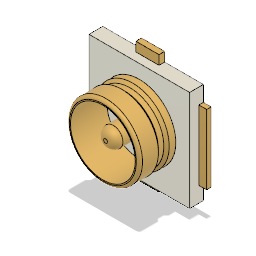
U.FL_Molex_MCRF_73412-0110_Vertical (Autodesk Fusion 360 design; units mm, degrees)
Autodesk Fusion 360 part; units mm, degrees
sketch "Sketch1" plane through (0, 0, 0) normal (0, 0, 1) x (1, 0, 0)
  line L0 (-1.3, 1.3) -> (1.3, 1.3)
  line L1 (1.3, 1.3) -> (1.3, -1.3)
  line L2 (1.3, -1.3) -> (-1.3, -1.3)
  line L3 (-1.3, -1.3) -> (-1.3, 1.3)
  line L4 (-1.3, -1) -> (-1, -1.3)
  line L5 (-1.3, -1) -> (-0.9678, -1) construction
  dimension "d1" = 2.6
  dimension "d2" = 2.6
  dimension "d3" = 1.3
  dimension "d4" = 1.3
  dimension "d5" = 45
  dimension "d7" = 1
  constraint horizontal L0
  constraint vertical L1
  constraint horizontal L2
  constraint vertical L3
  constraint horizontal L5
  constraint coincident L3 L4.start
  constraint coincident L2 L4.end
  measures "d1" distance of L0.start L2.end
  measures "d2" distance of L0.start L0.end
  measures "d3" distance of origin L3
  measures "d4" distance of origin L0
  measures "d5" angle of L4 L5
  measures "d7" vertical distance of origin L4.start
extrude "Extrude1" add sketch "Sketch1" along normal blind 0.36 contours L0 L1 L2 L3 L4
sketch "Sketch2" plane through (0, 1.3, 0) normal (0, 1, 0) x (-1, 0, 0)
  line L0 (-1.3, 0) -> (1.3, 0)
  line L1 (1.3, 0) -> (1.3, 0.36)
  line L2 (1.3, 0.36) -> (-1.3, 0.36)
  line L3 (-1.3, 0.36) -> (-1.3, 0)
  line L4 (-0.3, 0.15) -> (0.3, 0.15)
  line L5 (0.3, 0.15) -> (0.3, 0)
  line L6 (0.3, 0) -> (-0.3, 0)
  line L7 (-0.3, 0) -> (-0.3, 0.15)
  dimension "d10" = 0.6
  dimension "d11" = 0.3
  dimension "d12" = 0.15
  constraint horizontal L4
  constraint vertical L5
  constraint horizontal L6
  constraint vertical L7
  constraint coincident L0 L5.end
  measures "d10" distance of L4.start L4.end
  measures "d11" distance of origin L7
  measures "d12" distance of L4.start L6.end
extrude "Extrude2" add sketch "Sketch2" along normal blind 0.24 contours L0 L4 L5 L6 L7
sketch "Sketch3" plane through (0, -1.3, 0) normal (0, -1, 0) x (1, 0, 0)
  line L0 (-1, 0) -> (1.3, 0)
  line L1 (1.3, 0) -> (1.3, 0.36)
  line L2 (1.3, 0.36) -> (-1, 0.36)
  line L3 (-1, 0.36) -> (-1, 0)
  line L4 (-0.3, 0.15) -> (0.3, 0.15)
  line L5 (0.3, 0.15) -> (0.3, 0)
  line L6 (0.3, 0) -> (-0.3, 0)
  line L7 (-0.3, 0) -> (-0.3, 0.15)
  dimension "d15" = 0.6
  dimension "d16" = 0.3
  dimension "d17" = 0.15
  constraint horizontal L4
  constraint vertical L5
  constraint horizontal L6
  constraint vertical L7
  constraint coincident L0 L5.end
  measures "d15" distance of L4.start L4.end
  measures "d16" distance of origin L7
  measures "d17" distance of L4.start L6.end
extrude "Extrude3" add sketch "Sketch3" along normal blind 0.24 contours L0 L4 L5 L6 L7
sketch "Sketch4" plane through (1.3, 0, 0) normal (1, 0, 0) x (0, 0, -1)
  line L0 (0, -1.3) -> (0, 1.3)
  line L1 (0, 1.3) -> (-0.36, 1.3)
  line L2 (-0.36, 1.3) -> (-0.36, -1.3)
  line L3 (-0.36, -1.3) -> (0, -1.3)
  line L4 (-0.12, -0.9) -> (0, -0.9)
  line L5 (0, -0.9) -> (0, 0.9)
  line L6 (0, 0.9) -> (-0.12, 0.9)
  line L7 (-0.12, 0.9) -> (-0.12, -0.9)
  dimension "d20" = 1.8
  dimension "d21" = 0.9
  dimension "d22" = 0.12
  constraint horizontal L4
  constraint vertical L5
  constraint horizontal L6
  constraint vertical L7
  constraint coincident L0 L5.end
  measures "d20" distance of L4.start L6.end
  measures "d21" distance of origin L4
  measures "d22" distance of L4.start L4.end
extrude "Extrude4" add sketch "Sketch4" along normal blind 0.2 and the other way blind 2.8 contours L0 L4 L5 L6 L7
sketch "Sketch5" plane through (0, 0, 0) normal (0, 1, 0) x (1, 0, 0)
  line L0 (-0.945, -0.36) -> (-0.945, -1.22)
  line L1 (-0.865, -1.3) -> (-0.835, -1.3)
  line L2 (-0.835, -1.3) -> (-0.835, -0.36)
  line L3 (-1, -0.36) -> (1.3, -0.36)
  line L4 (-0.945, -0.81) -> (-0.875, -0.74)
  line L5 (-0.875, -0.74) -> (-0.875, -0.6)
  line L6 (-0.875, -0.6) -> (-0.945, -0.53)
  arc A0 (-0.945, -1.22) -> (-0.865, -1.3) centre (-0.865, -1.22) ccw
  line L7 (-0.05, -1.23) -> (0, -1.23)
  line L8 (0, -1.23) -> (0, -0.36)
  line L9 (0, -0.36) -> (-0.25, -0.36)
  line L10 (-0.25, -0.36) -> (-0.25, -1.03)
  arc A1 (-0.25, -1.03) -> (-0.05, -1.23) centre (-0.05, -1.03) ccw
  point P0 (-0.25, -1.23)
  dimension "d27" = 0.94
  dimension "d28" = 0.11
  dimension "d29" = 0.28
  dimension "d30" = 0.49
  dimension "d31" = 135
  dimension "d32" = 0.14
  dimension "d33" = 0.945
  dimension "d34" = 0.08
  dimension "d35" = 1.23
  dimension "d36" = 0.25
  dimension "d37" = 0.25
  dimension "d38" = 0.2
  constraint vertical L0
  constraint perpendicular L0 L1
  constraint perpendicular L1 L2
  constraint coincident L2.end L3
  constraint coincident L0 L4.start
  constraint parallel L0 L5
  constraint coincident L0 L6.end
  constraint perpendicular L4 L6
  constraint coincident L0.start L3
  constraint tangent L0 A0
  constraint tangent L1 A0
  constraint horizontal L7
  constraint vertical L8
  constraint horizontal L9
  constraint vertical L10
  constraint coincident L3 L8.end
  constraint coincident P0 L7
  constraint coincident P0 L10
  constraint tangent L7 A1
  constraint tangent L10 A1
  measures "d27" distance of L1.end L2.end
  measures "d28" distance of L0 L2
  measures "d29" distance of L4.start L6.end
  measures "d30" vertical distance of L1.end L4.start
  measures "d31" angle of L5 L6 L3.end
  measures "d32" distance of L4.end L5.end
  measures "d33" distance of origin L0
  measures "d34" radius of A0
  measures "d35" distance of origin L7
  measures "d36" distance of P0 L7.end
  measures "d37" distance of origin L10
  measures "d38" radius of A1
revolve "Revolve1" add sketch "Sketch5" angle 360 about axis through (0, 0, 1.75) along (0, 0, 1) contours L0 L1 L2 L3 L4 L5 L6 A0 | L3 L7 L8 L9 L10 A1
equation "d3 = d1 / 2"
equation "d4 = d2 / 2"
equation "d11 = d10 / 2"
equation "d16 = d15 / 2"
equation "d21 = d20 / 2"
equation "d33 = 1 mm - d28 / 2"
